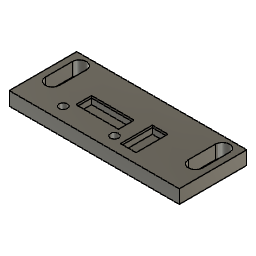
Mechanical Endstop Mount (Autodesk Fusion 360 design; units mm, degrees)
Autodesk Fusion 360 part; units mm, degrees
sketch "Sketch1" plane through (0, 0, 0) normal (0, 0, 1) x (1, 0, 0)
  line L0 (31.5, -12.5) -> (-31.5, -12.5)
  line L1 (-31.5, -12.5) -> (-31.5, 12.5)
  line L2 (-31.5, 12.5) -> (31.5, 12.5)
  line L3 (31.5, 12.5) -> (31.5, -12.5)
  line L4 (31.5, -12.5) -> (-31.5, 12.5) construction
  line L5 (-31.5, -12.5) -> (31.5, 12.5) construction
  circle A0 centre (-16.5, -7.5) radius 1.5
  circle A1 centre (2.5, -7.5) radius 1.5
  line L6 (-29.125, 8.5) -> (-29.125, -1.5)
  arc A2 (-29.125, -1.5) -> (-23.875, -1.5) centre (-26.5, -1.5) ccw
  line L7 (-23.875, -1.5) -> (-23.875, 8.5)
  arc A3 (-23.875, 8.5) -> (-29.125, 8.5) centre (-26.5, 8.5) ccw
  line L8 (-26.5, 8.5) -> (-26.5, -1.5) construction
  line L9 (29.125, -1.5) -> (29.125, 8.5)
  arc A4 (29.125, 8.5) -> (23.875, 8.5) centre (26.5, 8.5) ccw
  line L10 (23.875, 8.5) -> (23.875, -1.5)
  arc A5 (23.875, -1.5) -> (29.125, -1.5) centre (26.5, -1.5) ccw
  line L11 (26.5, -1.5) -> (26.5, 8.5) construction
  line L12 (-14.25, 0.75) -> (0.75, 0.75)
  line L13 (0.75, 0.75) -> (0.75, -4.25)
  line L14 (0.75, -4.25) -> (-14.25, -4.25)
  line L15 (-14.25, -4.25) -> (-14.25, 0.75)
  line L16 (-14.25, -1.75) -> (0.75, -1.75) construction
  line L17 (6.5, 2.5) -> (11.5, 2.5)
  line L18 (11.5, 2.5) -> (11.5, -8.5)
  line L19 (11.5, -8.5) -> (6.5, -8.5)
  line L20 (6.5, -8.5) -> (6.5, 2.5)
  line L21 (9, 2.5) -> (9, -8.5) construction
  line L22 (-6.75, 0.75) -> (-6.75, -4.25) construction
  dimension "d1" = 63
  dimension "d2" = 25
  dimension "d3" = 3
  dimension "d4" = 3
  dimension "d5" = 19
  dimension "d6" = 5
  dimension "d7" = 5
  dimension "d8" = 15
  dimension "d9" = 5.25
  dimension "d10" = 5.25
  dimension "d11" = 5
  dimension "d12" = 5
  dimension "d15" = 4
  dimension "d16" = 4
  dimension "d17" = 10
  dimension "d18" = 10
  dimension "d19" = 5
  dimension "d20" = 5.75
  dimension "d21" = 5
  dimension "d22" = 15
  dimension "d23" = 2.25
  dimension "d24" = 11
  dimension "d25" = 6.5
  dimension "d26" = 1
  constraint horizontal L0
  constraint perpendicular L0 L1
  constraint parallel L0 L2
  constraint parallel L1 L3
  constraint coincident L4 origin
  constraint coincident L5 origin
  constraint tangent L6 A2
  constraint tangent A2 L7
  constraint parallel L6 L7
  constraint tangent L7 A3
  constraint tangent L6 A3
  constraint vertical L8
  constraint tangent L9 A4
  constraint tangent A4 L10
  constraint parallel L9 L10
  constraint tangent L10 A5
  constraint tangent L9 A5
  constraint vertical L11
  constraint horizontal L12
  constraint vertical L13
  constraint horizontal L14
  constraint vertical L15
  constraint midpoint L15 L16.start
  constraint midpoint L13 L16.end
  constraint horizontal L17
  constraint vertical L18
  constraint horizontal L19
  constraint vertical L20
  constraint midpoint L17 L21.start
  constraint midpoint L19 L21.end
  constraint midpoint L12 L22.start
  constraint midpoint L14 L22.end
  constraint symmetric L12.start L12.end L22
  constraint coincident L18.end L19.start
  measures "d1" distance of L1.end L2.end
  measures "d2" distance of L0.end L1.end
  measures "d3" diameter of A0
  measures "d4" diameter of A1
  measures "d5" distance of A0.centre A1.centre
  measures "d6" distance of L0 A0.centre
  measures "d7" distance of L0 A1.centre
  measures "d8" distance of L1 A0.centre
  measures "d9" diameter of A2
  measures "d10" diameter of A4
  measures "d11" distance of L1 A2.centre
  measures "d12" distance of L3 A4.centre
  measures "d15" distance of L2 A3.centre
  measures "d16" distance of L2 A4.centre
  measures "d17" distance of A3.centre A2.centre
  measures "d18" distance of A5.centre A4.centre
  measures "d19" distance of L12.start L14.end
  measures "d20" vertical distance of A0.centre L16.start
  measures "d21" distance of L17.start L17.end
  measures "d22" distance of L12.start L12.end
  measures "d23" horizontal distance of A0.centre L14.end
  measures "d24" distance of L17.end L18.end
  measures "d25" horizontal distance of A1.centre L21.end
  measures "d26" vertical distance of A1.centre L19.end
extrude "Extrude1" add sketch "Sketch1" along normal blind 5 contours L0 L1 L2 L3 | L12 L13 L14 L15 | L17 L18 L19 L20
extrude "Extrude2" cut sketch "Sketch1" against normal blind 2.5 from surface at 5 contours L12 L13 L14 L15 | L17 L18 L19 L20
chamfer "Chamfer1" distance 0.4 angle 45 8 edges at (-6.75, 0.75, 5) (-14.25, -1.75, 5) (-6.75, -4.25, 5) (0.75, -1.75, 5) (9, 2.5, 5) (6.5, -3, 5) (11.5, -3, 5) (9, -8.5, 5)
equation "d7 = d6"
equation "d10 = d9"
equation "d12 = d11"
equation "d16 = d15"
equation "d18 = d17"
